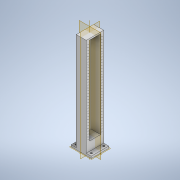
# Autodesk Inventor part: PushSupport
Saved by Autodesk Inventor 2021 (Build 250183000, 183)
## iProperties
Created: 2022-11-29
Part Number: PushSupport
Material: Generisch
Document SubType Name: Modeling
Designer: Elian
Density: 1 g/cm^3
Appearance: Vorgabe
Author: Elian
Autodesk Inventor part; units mm, degrees
sketch "Skizze1" plane through (0, 0, 0) normal (0, 0, 1) x (1, 0, 0)
  line L0 (-10, 4) -> (10, 4)
  line L1 (-20, 0) -> (20, 0)
  line L2 (20, 0) -> (20, 4)
  line L3 (20, 4) -> (-20, 4)
  line L4 (-20, 4) -> (-20, 0)
  line L5 (-10, 4) -> (10, 4)
  line L6 (10, 4) -> (10, 200)
  line L7 (10, 200) -> (-10, 200)
  line L8 (-10, 200) -> (-10, 4)
  point P0 (0, 0)
  dimension "d4" = 40
  dimension "d5" = 4
  dimension "d15" = 20
  dimension "d16" = 196
  constraints: 18 end point, 4 parallel, 3 horizontal, 2 collinear, 2 perpendicular
  measures "d4" distance of L3.end L2.end
  measures "d5" distance of L2.end L1.end
  measures "d15" distance of L7.end L6.end
  measures "d16" distance of L6.end L5.end
extrude "Extrusion1" add sketch "Skizze1" along normal mid plane 35
sketch "Skizze3" plane through (10, 4, 17.5) normal (1, 0, 0) x (0, 0, -1)
  line L0 (6.2495, 193) -> (28.7505, 193)
  line L1 (28.7505, 193) -> (28.7505, 18)
  line L2 (28.7505, 18) -> (6.2495, 18)
  line L3 (6.2495, 18) -> (6.2495, 193)
  line L4 (17.5, -44) -> (17.5, 236) projected
  line L5 (35, 196) -> (0, 196) projected
  line L6 (35, 196) -> (35, 0) projected
  line L7 (0, 0) -> (0, 196) projected
  point P0 (17.5, -4)
  dimension "d17" = 22.501
  dimension "d18" = 175
  dimension "d19" = 3
  dimension "d22" = 6.2495
  dimension "d27" = 6.2495
  constraints: 8 end point, 2 parallel, 1 horizontal, 1 perpendicular, 1 other
  measures "d17" distance of L0.start L0.end
  measures "d18" distance of L0.end L1.end
  measures "d19" distance between parallel lines of L5 L0
  measures "d22" distance between parallel lines of L6 L1
  measures "d27" distance between parallel lines of L7 L3
extrude "Extrusion3" cut sketch "Skizze3" against normal through all
sketch "Skizze4" plane through (10, 4, 17.5) normal (1, 0, 0) x (0, 0, -1)
  circle A0 centre (3.65, 186.5) radius 0.5
  line L0 (6.2495, 193) -> (28.7505, 193) projected
  line L1 (17.5, 159.9613) -> (17.5, 155.7748)
  circle A1 centre (31.35, 186.5) radius 0.5
  line L2 (17.5, -44) -> (17.5, 236) projected
  line L3 (6.2495, 18) -> (6.2495, 193) projected
  line L4 (28.7505, 193) -> (28.7505, 18) projected
  circle A2 centre (3.65, 181.5) radius 0.5
  circle A3 centre (31.35, 181.5) radius 0.5
  circle A4 centre (3.65, 176.5) radius 0.5
  circle A5 centre (31.35, 176.5) radius 0.5
  circle A6 centre (3.65, 171.5) radius 0.5
  circle A7 centre (31.35, 171.5) radius 0.5
  circle A8 centre (3.65, 166.5) radius 0.5
  circle A9 centre (31.35, 166.5) radius 0.5
  circle A10 centre (3.65, 161.5) radius 0.5
  circle A11 centre (31.35, 161.5) radius 0.5
  circle A12 centre (3.65, 156.5) radius 0.5
  circle A13 centre (31.35, 156.5) radius 0.5
  circle A14 centre (3.65, 151.5) radius 0.5
  circle A15 centre (31.35, 151.5) radius 0.5
  circle A16 centre (3.65, 146.5) radius 0.5
  circle A17 centre (31.35, 146.5) radius 0.5
  circle A18 centre (3.65, 141.5) radius 0.5
  circle A19 centre (31.35, 141.5) radius 0.5
  circle A20 centre (3.65, 136.5) radius 0.5
  circle A21 centre (31.35, 136.5) radius 0.5
  circle A22 centre (3.65, 131.5) radius 0.5
  circle A23 centre (31.35, 131.5) radius 0.5
  circle A24 centre (3.65, 126.5) radius 0.5
  circle A25 centre (31.35, 126.5) radius 0.5
  circle A26 centre (3.65, 121.5) radius 0.5
  circle A27 centre (31.35, 121.5) radius 0.5
  circle A28 centre (3.65, 116.5) radius 0.5
  circle A29 centre (31.35, 116.5) radius 0.5
  circle A30 centre (3.65, 111.5) radius 0.5
  circle A31 centre (31.35, 111.5) radius 0.5
  circle A32 centre (3.65, 106.5) radius 0.5
  circle A33 centre (31.35, 106.5) radius 0.5
  circle A34 centre (3.65, 101.5) radius 0.5
  circle A35 centre (31.35, 101.5) radius 0.5
  circle A36 centre (3.65, 96.5) radius 0.5
  circle A37 centre (31.35, 96.5) radius 0.5
  circle A38 centre (3.65, 91.5) radius 0.5
  circle A39 centre (31.35, 91.5) radius 0.5
  circle A40 centre (3.65, 86.5) radius 0.5
  circle A41 centre (31.35, 86.5) radius 0.5
  circle A42 centre (3.65, 81.5) radius 0.5
  circle A43 centre (31.35, 81.5) radius 0.5
  circle A44 centre (3.65, 76.5) radius 0.5
  circle A45 centre (31.35, 76.5) radius 0.5
  circle A46 centre (3.65, 71.5) radius 0.5
  circle A47 centre (31.35, 71.5) radius 0.5
  point P0 (17.5, -4)
  dimension "d23" = 1
  dimension "d24" = 6.5
  dimension "d25" = 27.7
  dimension "d26" = 22.501
  dimension "d30" = 5
  constraints: 48 centre point, 2 end point, 2 symmetric about line, 2 vertical, 93 other
  measures "d23" diameter of A0
  measures "d24" distance from line of L0 A0.centre
  measures "d25" distance of A0.centre A1.centre
  measures "d26" distance between parallel lines of L3 L4
  measures "d30" distance of A0.centre A2.centre
hole "Bohrung1" at (10, 190.5, 13.85) direction (-1, 0, 0) diameter 0.7294 depth 8 tip angle 118 thread size "M1x0.25" class "6H" standard "ISO Metric profile"
pattern_linear "Rechteckige Anordnung1" count 34 spacing 5 along (0, -1, 0) count 2 spacing 27.7 along (0, 0, -1) of "Bohrung1"
sketch "Skizze5" plane through (10, 4, 17.5) normal (0, 1, 0) x (1, 0, 0)
  point P0 (-10, 17.5)
  point P1 (5, 5)
  point P2 (5, 30)
hole "Bohrung2" at (15, 4, 12.5) at (15, 4, -12.5) direction (0, -1, 0) diameter 3.6881 depth 13 tip angle 118 thread size "M4.5x0.75" class "6H" standard "ISO Metric profile"
sketch "Skizze6" plane through (-20, 4, 17.5) normal (0, 1, 0) x (1, 0, 0)
  point P0 (20, 17.5)
  point P1 (5, 30)
  point P2 (5, 5)
hole "Bohrung3" at (-15, 4, -12.5) at (-15, 4, 12.5) direction (0, -1, 0) diameter 3.6881 depth 13 tip angle 118 thread size "M4.5x0.75" class "6H" standard "ISO Metric profile"
